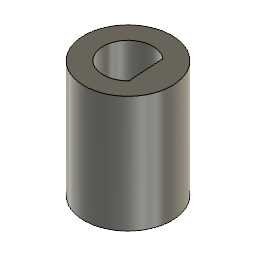
encoder_coupler (Autodesk Fusion 360 design; units mm, degrees)
Autodesk Fusion 360 part; units mm, degrees
sketch "Sketch5" plane through (0, 0, 0) normal (0, 0, 1) x (1, 0, 0)
  circle A0 centre (0, 0) radius 7.5
  line L0 (2.5, 2.0767) -> (2.5, -2.0767)
  arc A1 (2.5, 2.0767) -> (2.5, -2.0767) centre (0, 0) ccw
  dimension "d22" = 15
  dimension "d29" = 6.5
  dimension "d30" = 2.5
  constraint coincident A0.centre A1.centre
  constraint vertical L0
  measures "d22" diameter of A0
  measures "d29" diameter of A1
  measures "d30" distance of A0.centre L0
extrude "Extrude5" add sketch "Sketch5" along normal blind 10
sketch "Sketch6" plane through (0, 0, 10) normal (0, 0, 1) x (-1, 0, 0)
  circle A0 centre (0, 0) radius 7.5
  circle A1 centre (0, 0) radius 7.5
  arc A2 (-2.5, -2.0767) -> (-2.5, 2.0767) centre (0, 0) ccw
  line L0 (-2.5, -2.0767) -> (-2.5, 2.0767)
  line L1 (-2.7005, -3.2818) -> (-3.0882, 2.9198)
  arc A3 (-2.7005, -3.2818) -> (-3.0882, 2.9198) centre (0, 0) ccw
  dimension "d31" = 8.5
  dimension "d32" = 2.9
  constraint concentric A1 A3
  measures "d31" diameter of A3
  measures "d32" distance of A0.centre L1
extrude "Extrude6" add sketch "Sketch6" along normal blind 10 contours A0 A1
